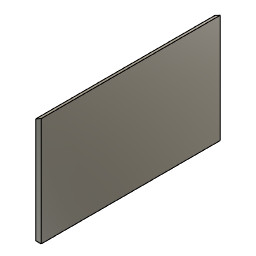
front1-bas v2 (Autodesk Fusion 360 design; units mm, degrees)
Autodesk Fusion 360 part; units mm, degrees
note: some values were not read from the file. Set by a fixed rule: which sketch regions a step uses.
sketch "Esquisse1" plane through (0, 0, 0) normal (0, 1, 0) x (1, 0, 0)
  line L0 (0, 0) -> (4, 0)
  line L1 (4, 0) -> (4, -80)
  line L2 (0, -77.8597) -> (0, 0)
  line L3 (0, -77.8597) -> (4, -80)
  dimension "d1" = 4
  dimension "d5" = 61.85
  constraint horizontal L0
  constraint vertical L1
  constraint vertical L2
  constraint coincident L0.start L2.end
  measures "d1" distance of L0.start L0.end
  measures "d5" angle of L1 L3
extrude "Extrusion1" add sketch "Esquisse1" along normal blind 132
